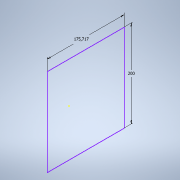
# Autodesk Inventor part: PlatteAußenGross
Saved by Autodesk Inventor 2020.3 (Build 243373010, 373A)
## iProperties
Created: 2021-02-12
Part Number: PlatteAußenGross
Material: Generisch
Document SubType Name: Modeling
Designer: Stefan
Density: 1 g/cm^3
Appearance: Vorgabe
Author: Stefan
Autodesk Inventor part; units mm, degrees
ref_plane "YZ Plane" through (0, 0, 0) normal (1, 0, 0) x (0, 1, 0)
ref_plane "XZ Plane" through (0, 0, 0) normal (0, 1, 0) x (-1, 0, 0)
ref_plane "XY Plane" through (0, 0, 0) normal (0, 0, 1) x (1, 0, 0)
sketch "Skizze1" plane through (0, 0, 0) normal (1, 0, 0) x (0, 1, 0)
  line L0 (-106.6709, 345.5) -> (93.3291, 345.5)
  line L1 (93.3291, 345.5) -> (93.3291, -126.054)
  line L2 (93.3291, -126.054) -> (-106.6709, -126.054)
  line L3 (-106.6709, -126.054) -> (-106.6709, 345.5)
  point P0 (0, 0)
  dimension "d0" = 200
  dimension "d1" = 471.554
  constraints: 8 end point, 2 parallel, 1 horizontal, 1 perpendicular
  measures "d0" distance of L1.end L2.end
  measures "d1" distance of L0.end L1.end
extrude "Extrusion1" add sketch "Skizze1" along normal blind 10
